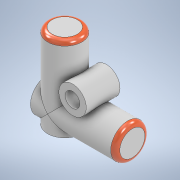
# Autodesk Inventor part: Union Elbow 1-8 KQ2L01-00A SMC
Saved by Autodesk Inventor 2021 (Build 250183000, 183)
## iProperties
Created: 2020-07-15
Part Number: Union Elbow 1-8 KQ2L01-00A SMC
Material: Generic
Document SubType Name: Modeling
Designer: jgray
Density: 1 g/cm^3
Appearance: Default
Author: jgray
Autodesk Inventor part; units mm, degrees
ref_plane "YZ Plane" through (0, 0, 0) normal (1, 0, 0) x (0, 1, 0)
ref_plane "XZ Plane" through (0, 0, 0) normal (0, 1, 0) x (-1, 0, 0)
ref_plane "XY Plane" through (0, 0, 0) normal (0, 0, 1) x (1, 0, 0)
sketch "Sketch1" plane through (0, 0, 0) normal (0, 1, 0) x (-1, 0, 0)
  circle A0 centre (0, 0) radius 3.75
  dimension "d0" = 7.5
  constraints: 1 centre point, 1 coincident
  measures "d0" diameter of A0
extrude "Extrusion1" add sketch "Sketch1" along normal blind 18.4
sketch "Sketch2" plane through (0, 0, 0) normal (1, 0, 0) x (0, 1, 0)
  circle A0 centre (3.75, 0) radius 3.75
  line L0 (0, -3.75) -> (0, 3.75) projected
  point P0 (0, 0)
  dimension "d3" = 7.5
  constraints: 1 centre point, 1 tangent
  measures "d3" diameter of A0
extrude "Extrusion2" add sketch "Sketch2" along normal blind 14.8 and the other way blind 3.75
sketch "Sketch3" plane through (0, 0, 0) normal (0, 0, 1) x (1, 0, 0)
  line L0 (17.8168, 3.75) -> (-11.5413, 3.75) construction
  line L1 (0, 19.7284) -> (0, -6.0231) construction
  line L2 (0, 3.75) -> (0, 3.75) construction
  line L3 (0, 3.75) -> (-3.75, 7.5) construction
  line L4 (-3.75, 7.5) -> (0, 3.75) construction
  line L5 (3.75, 18.4) -> (-3.75, 18.4) construction
  line L6 (0, 3.75) -> (3.75, 0) construction
  line L7 (0, 3.75) -> (0, 3.75) construction
  line L8 (3.75, 0) -> (0, 3.75) construction
  line L9 (14.8, 0) -> (14.8, 7.5) construction
  circle A0 centre (5.4, 9.15) radius 1.6
  circle A1 centre (5.4, 9.15) radius 3
  point P0 (0, 0)
  point P1 (0, 18.4)
  point P2 (14.8, 3.75)
  dimension "d8" = 5.4
  dimension "d9" = 5.4
  dimension "d10" = 3.2
  dimension "d11" = 6
  constraints: 4 end point, 2 centre point, 2 coincident, 2 midpoint, 2 point on line, 1 horizontal, 1 vertical
  measures "d8" distance from line of point (5.4, 9.15) L0
  measures "d9" distance from line of point (5.4, 9.15) L1
  measures "d10" diameter of A0
  measures "d11" diameter of A1
extrude "Extrusion3" add sketch "Sketch3" along normal mid plane 7.4
fillet "Fillet1" radius 1 2 edges at (3.75, 18.4, 0) (14.8, 0, 0)
body "Solid1"
